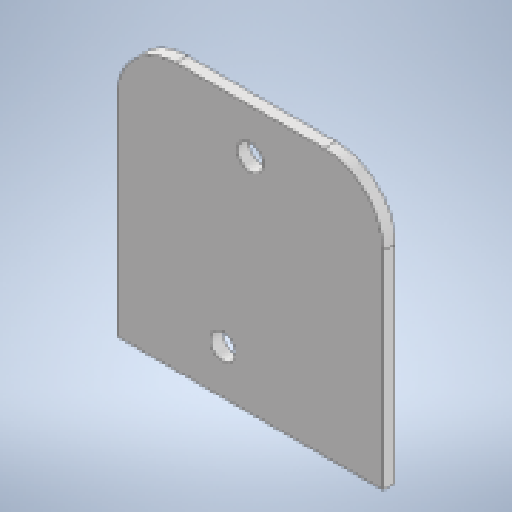
# Autodesk Inventor part: Ухо на стойку_CPY
Saved by Autodesk Inventor 2025 (Build 290162010, 162A)
## iProperties
Created: 2024-06-15
Part Number: Ухо на стойку_CPY
Material: Generic
Document SubType Name: Sheet Metal
Designer: admin
Density: 1 g/cm^3
Sheet Metal Rule: Default
Appearance: Default
Author: admin
Autodesk Inventor part; units mm, degrees
ref_plane "YZ Plane" through (0, 0, 0) normal (1, 0, 0) x (0, 1, 0)
ref_plane "XZ Plane" through (0, 0, 0) normal (0, 1, 0) x (-1, 0, 0)
ref_plane "XY Plane" through (0, 0, 0) normal (0, 0, 1) x (1, 0, 0)
sketch "Sketch1" plane through (0, 0, 0) normal (0, 1, 0) x (-1, 0, 0)
  line L0 (90, 90) -> (-90, 90)
  line L1 (-90, 90) -> (-90, -90)
  line L2 (-90, -90) -> (90, -90)
  line L3 (90, -90) -> (90, 90)
  point P0 (0, 0)
  point P1 (0, 90)
  point P2 (90, 0)
  dimension "d0" = 180
  dimension "d1" = 180
  measures "d0" distance of L0.start L0.end
  measures "d1" distance of L2.end L0.start
extrude "Plate1" add sketch "Sketch1" along normal mid plane 8
sketch "Sketch2" plane through (0, -4, 0) normal (0, -1, 0) x (1, 0, 0)
  line L0 (0, 60) -> (-18.2401, -60) construction
  line L1 (-90, -90) -> (-90, 90) projected
  line L2 (90, 90) -> (90, -90) projected
  point P0 (0, 0)
  point P1 (-9.12, 0)
  point P2 (-90, 0)
  dimension "d15" = 60
  constraints: 2 end point, 1 coincident, 1 horizontal alignment, 1 midpoint, 1 vertical alignment, 2 other
  measures "d15" distance of point (0, 0) L0.start
hole "Hole1" at (0, -4, 60) at (-18.2401, -4, -60) direction (0, 1, 0) diameter 17 end through all
fillet "Fillet1" radius 40 2 edges at (90, 0, 90) (-90, 0, 90)
equation "\"d1\" = d0"
equation "\"d8\" = Thickness"
equation "\"d2\" = Thickness"
equation "\"BendRadius\" = Thickness"
equation "\"BendReliefWidth\" = Thickness"
equation "\"BendReliefDepth\" = 0.5 * Thickness"
equation "\"CornerReliefSize\" = 4 * Thickness"
equation "\"MinimumRemnant\" = 2 * Thickness"
equation "\"TransitionRadius\" = BendRadius"
equation "\"JacobiRadiusSize\" = BendRadius"
equation "\"GapSize\" = Thickness"
equation "\"Thickness\" = 8"
body "Solid1"
